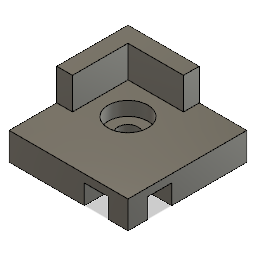
universeel voedingblokje v1 (Autodesk Fusion 360 design; units mm, degrees)
Autodesk Fusion 360 part; units mm, degrees
sketch "Sketch1" plane through (0, 0, 0) normal (0, 1, 0) x (1, 0, 0)
  line L0 (0, 0) -> (30, 0)
  line L1 (30, 0) -> (30, -30)
  line L2 (30, -30) -> (0, -30)
  line L3 (0, -30) -> (0, 0)
  dimension "d1" = 30
  dimension "d2" = 30
  constraint horizontal L0
  constraint vertical L1
  constraint horizontal L2
  constraint vertical L3
  constraint coincident L0.start L3.end
  measures "d1" distance of L0.start L0.end
  measures "d2" distance of L0.start L2.end
extrude "Extrude1" add sketch "Sketch1" along normal blind 7
sketch "Sketch2" plane through (0, 7, 0) normal (0, 1, 0) x (-1, 0, 0)
  line L0 (0, 30) -> (-30, 30)
  line L1 (-30, 30) -> (-30, 0)
  line L2 (-18, 0) -> (-18, 4)
  line L3 (-18, 4) -> (-4, 4)
  line L4 (-4, 4) -> (-4, 18)
  line L5 (-4, 18) -> (0, 18)
  line L6 (0, 18) -> (0, 0)
  line L7 (0, 0) -> (-18, 0)
  dimension "d9" = 18
  dimension "d10" = 18
  dimension "d11" = 4
  dimension "d12" = 4
  constraint vertical L2
  constraint perpendicular L2 L3
  constraint perpendicular L3 L4
  constraint perpendicular L4 L5
  constraint coincident L6.end L7.start
  constraint perpendicular L5 L6
  constraint perpendicular L2 L7
  measures "d9" distance of L5 L7
  measures "d10" distance of L2 L6
  measures "d11" distance of L2.start L2.end
  measures "d12" distance of L4.end L5.end
extrude "Extrude2" add sketch "Sketch2" along normal blind 8
sketch "Sketch3" plane through (0, 0, 0) normal (0, 0, -1) x (-1, 0, 0)
  line L0 (-30, 0) -> (0, 0)
  line L1 (0, 0) -> (0, 15)
  line L2 (0, 15) -> (-18, 15)
  line L3 (-18, 15) -> (-18, 7)
  line L4 (-18, 7) -> (-30, 7)
  line L5 (-30, 7) -> (-30, 0)
  line L6 (-25, 0) -> (-19, 0)
  line L7 (-19, 0) -> (-19, 5)
  line L8 (-19, 5) -> (-25, 5)
  line L9 (-25, 5) -> (-25, 0)
  dimension "d13" = 6
  dimension "d14" = 5
  dimension "d15" = 5
  constraint horizontal L6
  constraint vertical L7
  constraint horizontal L8
  constraint vertical L9
  constraint coincident L0 L6.start
  measures "d13" distance of L6.start L6.end
  measures "d14" distance of L6 L8
  measures "d15" distance of L5 L9
extrude "Extrude3" cut sketch "Sketch3" against normal through all contours L0 L6 L7 L8 L9
sketch "Sketch4" plane through (0, 7, 0) normal (0, 1, 0) x (-1, 0, 0)
  line L0 (-4, 18) -> (0, 18)
  line L1 (0, 18) -> (0, 30)
  line L2 (0, 30) -> (-30, 30)
  line L3 (-30, 30) -> (-30, 0)
  line L4 (-30, 0) -> (-18, 0)
  line L5 (-18, 0) -> (-18, 4)
  line L6 (-18, 4) -> (-4, 4)
  line L7 (-4, 4) -> (-4, 18)
  line L8 (-19, 0) -> (-19, 30)
  point P0 (-12, 12)
  dimension "d18" = 8
  dimension "d28" = 8
  measures "d18" distance of L6 P0
  measures "d28" distance of L7 P0
hole "Hole1" at (12, 7, 12) direction (0, -1, 0) diameter 5 end through all counterbore diameter 10 counterbore depth 3.5
sketch "Sketch5" plane through (0, 0, 0) normal (-1, 0, 0) x (0, 0, 1)
  line L0 (0, 0) -> (30, 0)
  line L1 (30, 0) -> (30, 7)
  line L2 (30, 7) -> (18, 7)
  line L3 (18, 7) -> (18, 15)
  line L4 (18, 15) -> (0, 15)
  line L5 (0, 15) -> (0, 0)
  line L6 (25, 0) -> (19, 0)
  line L7 (19, 0) -> (19, 5)
  line L8 (19, 5) -> (25, 5)
  line L9 (25, 5) -> (25, 0)
  dimension "d24" = 6
  dimension "d25" = 5
  dimension "d26" = 5
  constraint horizontal L6
  constraint vertical L7
  constraint horizontal L8
  constraint vertical L9
  constraint coincident L0 L6.start
  measures "d24" distance of L6.start L6.end
  measures "d25" distance of L6.end L7.end
  measures "d26" distance of L1 L9
extrude "Extrude4" cut sketch "Sketch5" against normal through all contours L0 L6 L7 L8 L9
equation "d9 = d10"
